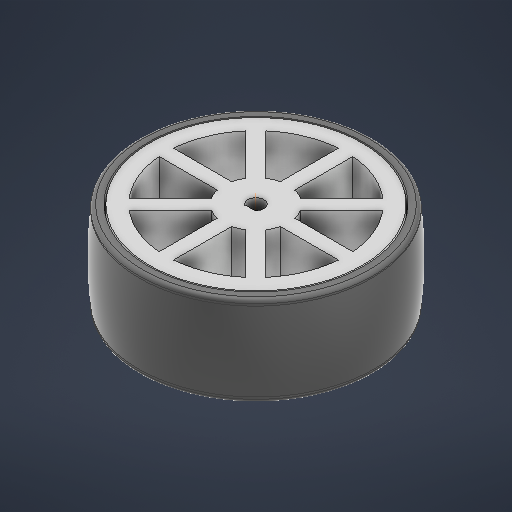
# Autodesk Inventor part: wheel
Saved by Autodesk Inventor 2027 (Build 310192000, 192)
## iProperties
Created: 2026-05-11
Part Number: wheel
Material: Generic
Document SubType Name: Modeling
Designer: maksi
Density: 1 g/cm^3
Appearance: Default
Author: maksi
Autodesk Inventor part; units mm, degrees
ref_plane "YZ Plane" through (0, 0, 0) normal (1, 0, 0) x (0, 1, 0)
ref_plane "XZ Plane" through (0, 0, 0) normal (0, 1, 0) x (-1, 0, 0)
sketch "Sketch1" plane through (0, 0, 0) normal (0, 1, 0) x (-1, 0, 0)
  circle A0 centre (-0.0227, 0.0341) radius 32.5
  arc A1 (-1.3456, 1.5341) -> (1.3002, 1.5341) centre (-0.0227, 0.0341) ccw
  line L0 (1.3002, 1.5341) -> (-1.3456, 1.5341)
  arc A2 (-1.4191, 1.7341) -> (1.3737, 1.7341) centre (-0.0227, 0.0341) ccw
  line L1 (-1.4191, 1.7341) -> (1.3737, 1.7341)
  circle A3 centre (-0.0227, 0.0341) radius 29.5
  circle A4 centre (-0.0227, 0.0341) radius 29.875
  circle A5 centre (1.3737, 1.7341) radius 0.1
  circle A6 centre (-1.4191, 1.7341) radius 0.1
  point P0 (0, 0)
  point P1 (-1.4949, 1.6688)
  point P2 (-1.3191, 1.7341)
  point P3 (1.2737, 1.7341)
  point P4 (1.4495, 1.6688)
  dimension "d0" = 65
  dimension "d1" = 0.2
  dimension "d2" = 59
  dimension "d3" = 59.75
  dimension "d9" = 0.2
  dimension "d10" = 0.2
  constraints: 7 centre point, 4 coincident, 4 end point, 4 point on circle, 1 other
  measures "d0" diameter of A0
  measures "d1" radial gap between concentric circles of A1 A2
  measures "d2" diameter of A3
  measures "d3" diameter of A4
  measures "d9" diameter of A5
  measures "d10" diameter of A6
extrude "Extrusion1" add sketch "Sketch1" along normal blind 25 contours A3
extrude "Extrusion2" add sketch "Sketch1" along normal blind 25 separate body contours A0
fillet "Fillet1" radius 1 2 edges at (32.5227, 25, 0.0341) (32.5227, 0, 0.0341)
sketch "Sketch2" plane through (0.0227, 25, 0.0341) normal (0, 1, 0) x (1, 0, 0)
  circle A0 centre (-0.0227, 0.0341) radius 9
  circle A1 centre (-0.0227, 0.0341) radius 25
  line L0 (-18.0392, 20.8195) -> (20.8516, -18.0714)
  line L1 (20.8516, -18.0714) -> (18.0232, -20.8998)
  line L2 (18.0232, -20.8998) -> (-20.8677, 17.9911)
  line L3 (-20.8677, 17.9911) -> (-18.0392, 20.8195)
  line L4 (27.4773, -1.9659) -> (-27.5227, 2.0341) construction
  line L5 (-27.5227, -1.9659) -> (27.4773, 2.0341) construction
  line L6 (1.9773, -27.4659) -> (-2.0227, -27.4659)
  line L7 (-2.0227, -27.4659) -> (-2.0227, 27.5341)
  line L8 (-2.0227, 27.5341) -> (1.9773, 27.5341)
  line L9 (1.9773, 27.5341) -> (1.9773, -27.4659)
  line L10 (1.9773, -27.4659) -> (-2.0227, 27.5341) construction
  line L11 (-2.0227, -27.4659) -> (1.9773, 27.5341) construction
  line L12 (27.4773, -1.9659) -> (-27.5227, -1.9659)
  line L13 (-27.5227, -1.9659) -> (-27.5227, 2.0341)
  line L14 (-27.5227, 2.0341) -> (27.4773, 2.0341)
  line L15 (27.4773, 2.0341) -> (27.4773, -1.9659)
  line L16 (27.4773, -1.9659) -> (-27.5227, 2.0341) construction
  line L17 (-27.5227, -1.9659) -> (27.4773, 2.0341) construction
  line L18 (-20.8195, -18.0392) -> (18.0714, 20.8516)
  line L19 (18.0714, 20.8516) -> (20.8998, 18.0232)
  line L20 (20.8998, 18.0232) -> (-17.9911, -20.8677)
  line L21 (-17.9911, -20.8677) -> (-20.8195, -18.0392)
  point P0 (1.9773, -8.7409)
  point P1 (1.9773, -24.8858)
  point P2 (16.1519, -19.0285)
  point P3 (4.7313, -7.6079)
  point P4 (24.8972, -1.9659)
  point P5 (8.7523, -1.9659)
  point P6 (7.5733, -4.793)
  point P7 (18.9851, -16.2049)
  point P8 (19.0607, 16.1841)
  point P9 (7.6366, 4.76)
  point P10 (8.7523, 2.0341)
  point P11 (24.8972, 2.0341)
  point P12 (4.8321, 7.6124)
  point P13 (16.2407, 19.021)
  point P14 (1.9773, 24.9539)
  point P15 (1.9773, 8.809)
  point P16 (-2.0227, 8.809)
  point P17 (-2.0227, 24.9539)
  point P18 (-16.2616, 19.0419)
  point P19 (-4.8498, 7.6301)
  point P20 (-24.9426, 2.0341)
  point P21 (-8.7977, 2.0341)
  point P22 (-7.6647, 4.7881)
  point P23 (-19.0853, 16.2087)
  point P24 (-19.0096, -16.2293)
  point P25 (-7.601, -4.8208)
  point P26 (-8.7977, -1.9659)
  point P27 (-24.9426, -1.9659)
  point P28 (-4.7487, -7.6253)
  point P29 (-16.1728, -19.0493)
  point P30 (-2.0227, -24.8858)
  point P31 (-2.0227, -8.7409)
  dimension "d11" = 18
  dimension "d12" = 50
  dimension "d13" = 55
  dimension "d14" = 4
  dimension "d15" = 4
  dimension "d16" = 55
  constraints: 44 end point, 8 parallel, 6 midpoint, 4 perpendicular, 2 centre point, 2 coincident, 2 horizontal
  measures "d11" diameter of A0
  measures "d12" diameter of A1
  measures "d13" distance of L1.end L2.end
  measures "d14" distance of L0.end L1.end
  measures "d15" distance of L7.end L8.end
  measures "d16" distance of L6.end L7.end
extrude "Extrusion3" cut sketch "Sketch2" against normal blind 25 contours A0 L20 A1 L14 | L12 A1 L0 A0 | A0 L9 A1 L18 | L2 A1 L9 A0 | A0 L0 A1 L7 | L7 A1 L20 A0 | A0 L14 A1 L2 | L18 A1 L12 A0 bodies 1
ref_plane "Work Plane1" through (-24.9199, 25, 0) normal (0, 0, 1) x (1, 0, 0)
sketch "Sketch3" plane through (-24.9199, 25, 0) normal (0, 0, 1) x (1, 0, 0)
  line L0 (-7.5574, -24) -> (-7.5574, -1) projected
  line L1 (57.4426, -24) -> (57.4426, -1) projected
  line L2 (57.4426, -1) -> (-7.5574, -1)
  line L3 (-7.5574, -1) -> (-7.5574, -24)
  line L4 (-7.5574, -24) -> (57.4426, -24)
  line L5 (57.4426, -24) -> (57.4426, -1)
  arc A0 (-7.5574, -1) -> (-7.5574, -24) centre (92.85, -12.5) ccw
  line L6 (-7.5574, -1) -> (57.4426, -24) construction
  line L7 (-7.5574, -24) -> (57.4426, -1) construction
  line L8 (26.4148, -25) -> (26.4148, 0) construction
  line L9 (26.4148, -13.0209) -> (26.4148, -1) construction
  line L10 (26.4148, -13.0209) -> (26.4148, -24) construction
  line L11 (24.9199, -30) -> (24.9199, 5) projected
  point P0 (24.9199, -25)
  constraints: 16 end point, 7 point on line, 2 parallel, 2 perpendicular, 2 point on circle, 1 centre point
revolve "Revolution1" add sketch "Sketch3" angle 360 about axis through (0, -10, 0) along (0, 1, 0) separate body contours A0 L0
extrude "Extrusion4" add sketch "Sketch1" along normal blind 7.5 contours L0 A1 | L1 A6 A2 | A2 A6 L1 | A6 L1 A5 A2 | A5 L1 A2 | A2 L1 A5 bodies 1
combine bodies "Combine1" operation type add bodies to combine 3 2
